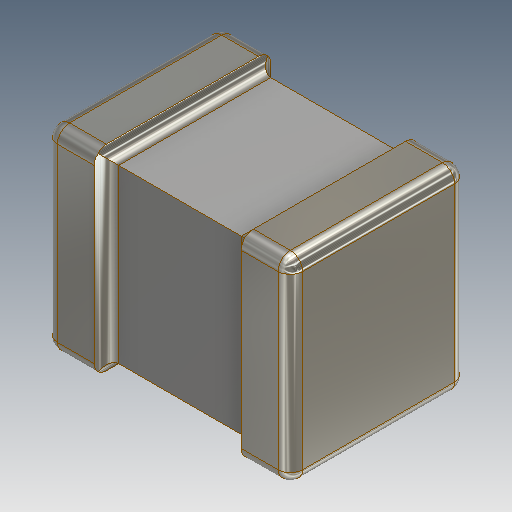
# Autodesk Inventor part: 1007
Saved by Autodesk Inventor 2017 (Build 210142000, 142)
## iProperties
Created: 2015-10-12
Part Number: 1007
Material: ABS Plastic
Document SubType Name: Modeling
Designer: Sawaiz
Density: 1.06 g/cm^3
Appearance: Smooth - Off-White
Author: Sawaiz
Autodesk Inventor part; units mm, degrees
ref_plane "YZ Plane" through (0, 0, 0) normal (1, 0, 0) x (0, 1, 0)
ref_plane "XZ Plane" through (0, 0, 0) normal (0, 1, 0) x (-1, 0, 0)
ref_plane "XY Plane" through (0, 0, 0) normal (0, 0, 1) x (1, 0, 0)
sketch "Sketch1" plane through (0, 0, 0) normal (0, 0, 1) x (1, 0, 0)
  line L0 (-0.9, -1.25) -> (0.9, -1.25)
  line L1 (0.9, -1.25) -> (0.9, 1.25)
  line L2 (0.9, 1.25) -> (-0.9, 1.25)
  line L3 (-0.9, 1.25) -> (-0.9, -1.25)
  line L4 (-0.9, -1.25) -> (0.9, 1.25) construction
  line L5 (0.9, -1.25) -> (-0.9, 1.25) construction
  point P0 (0, 0)
  dimension "d0" = 1.8
  dimension "d1" = 2.5
  constraints: 12 end point, 2 midpoint, 2 parallel, 1 horizontal, 1 perpendicular
  measures "d0" distance of L2.end L1.end
  measures "d1" distance of L1.end L0.end
extrude "Extrusion1" add sketch "Sketch1" along normal mid plane 2
sketch "Sketch2" plane through (0, 0, 1) normal (0, 0, 1) x (1, 0, 0)
  line L0 (-0.9, -1.25) -> (0.9, -1.25) projected
  line L1 (0.9, -1.25) -> (0.9, 1.25) projected
  line L2 (0.9, 1.25) -> (-0.9, 1.25) projected
  line L3 (-0.9, 1.25) -> (-0.9, -1.25) projected
  line L4 (0.9, 0.75) -> (-0.9, 0.75)
  line L5 (-0.9, 0.75) -> (-0.9, -0.75)
  line L6 (-0.9, -0.75) -> (0.9, -0.75)
  line L7 (0.9, -0.75) -> (0.9, 0.75)
  line L8 (0.9, 0.75) -> (-0.9, -0.75) construction
  line L9 (-0.9, 0.75) -> (0.9, -0.75) construction
  point P0 (0, 0)
  dimension "d4" = 0.5
  constraints: 12 end point, 2 midpoint, 2 parallel, 1 horizontal, 1 perpendicular, 1 point on line
  measures "d4" distance between parallel lines of L0 L6
extrude "Extrusion2" cut sketch "Sketch2" against normal blind 0.125 contours L3 L4 L1 L6
mirror "Mirror1" about plane through (0, 0, 0) normal (0, 0, 1) of "Extrusion2"
sketch "Sketch3" plane through (0.9, 1.25, 1) normal (1, 0, 0) x (0, 0, -1)
  line L0 (2, -2) -> (1.875, -2) projected
  line L1 (1.875, -2) -> (1.875, -0.5) projected
  line L2 (1.875, -0.5) -> (2, -0.5) projected
  line L3 (2, 0) -> (2, -0.5) projected
  line L4 (2, 0) -> (0, 0) projected
  line L5 (0, -0.5) -> (0, 0) projected
  line L6 (0, -0.5) -> (0.125, -0.5) projected
  line L7 (0.125, -0.5) -> (0.125, -2) projected
  line L8 (0.125, -2) -> (0, -2) projected
  line L9 (0, -2.5) -> (0, -2) projected
  line L10 (2, -2.5) -> (0, -2.5) projected
  line L11 (2, -2) -> (2, -2.5) projected
  line L12 (1.875, -2) -> (0.125, -2)
  line L13 (0.125, -2) -> (0.125, -0.5)
  line L14 (0.125, -0.5) -> (1.875, -0.5)
  line L15 (1.875, -0.5) -> (1.875, -2)
  line L16 (1.875, -2) -> (0.125, -0.5) construction
  line L17 (0.125, -2) -> (1.875, -0.5) construction
  point P0 (1, -1.25)
  constraints: 12 end point, 2 midpoint, 2 parallel, 1 horizontal, 1 perpendicular
extrude "Extrusion3" cut sketch "Sketch3" against normal blind 0.125 contours L12 L7 L14 L1
mirror "Mirror2" about plane through (0, 0, 0) normal (1, 0, 0) of "Extrusion3"
fillet "Fillet1" radius 0.125 24 edges at (0, -0.75, 0.875) (0.9, 1, 1) (0, 1.25, 1) (0.9, 1.25, 0) (0, 1.25, -1) (0.9, 1, -1) (0.9, -1, -1) (0.9, -1, 1) (0.775, -0.75, 0) (-0.9, -1, 1) (-0.9, 1, 1) (-0.9, 1.25, 0) (-0.9, 1, -1) (-0.9, -1, -1) (-0.9, -1.25, 0) (0, -1.25, 1) (0, -1.25, -1) (-0.775, -0.75, 0) (0, 0.75, 0.875) (-0.775, 0.75, 0) (0, 0.75, -0.875) (0, -0.75, -0.875) (0.775, 0.75, 0) (0.9, -1.25, 0)
equation "\"d0\" = width"
equation "\"d1\" = length"
equation "\"d2\" = height"
equation "\"d4\" = padLength"
equation "\"d5\" = 0.0625 * height"
equation "\"d7\" = 0.0625 * height"
equation "\"d9\" = 0.0625 * height"
equation "\"length\" = 2.5"
equation "\"padLength\" = 0.5"
equation "\"width\" = 1.8"
equation "\"height\" = 2"
body "Solid1"
